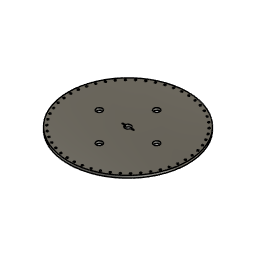
axe central v11 (Autodesk Fusion 360 design; units mm, degrees)
Autodesk Fusion 360 part; units mm, degrees
sketch "Esquisse1" plane through (0, 0, 0) normal (0, 0, 1) x (1, 0, 0)
  line L0 (-0.8543, -2.161) -> (-1.1188, -2.036)
  line L1 (1.1236, 2.043) -> (1.3703, 1.886)
  line L2 (-1.3655, -1.88) -> (-1.4051, -1.847)
  line L3 (-0.2892, -2.306) -> (-0.5764, -2.251)
  line L4 (-0.8543, 2.167) -> (-0.5764, 2.257)
  line L5 (1.4099, -1.847) -> (1.3703, -1.88)
  line L6 (-1.4051, 1.853) -> (-1.3655, 1.886)
  line L7 (1.4099, -0.321) -> (1.4099, -1.847)
  line L8 (1.3703, 1.886) -> (1.4099, 1.853)
  line L9 (-0.5764, -2.251) -> (-0.8543, -2.161)
  line L10 (-1.4051, -1.847) -> (-1.4051, -0.321)
  line L11 (0.0024, 2.331) -> (0.2941, 2.312)
  line L12 (-1.3655, 1.886) -> (-1.1188, 2.043)
  line L13 (-1.1188, 2.043) -> (-0.8543, 2.167)
  line L14 (1.4099, 1.853) -> (1.4099, 0.327)
  line L15 (4.9099, 0.327) -> (4.9099, -0.321)
  line L16 (0.0024, -2.324) -> (-0.2892, -2.306)
  line L17 (-4.9051, -0.321) -> (-4.9051, 0.327)
  line L18 (0.5813, -2.251) -> (0.2941, -2.306)
  line L19 (-0.5764, 2.257) -> (-0.2892, 2.312)
  line L20 (0.8591, 2.167) -> (1.1236, 2.043)
  line L21 (1.3703, -1.88) -> (1.1236, -2.036)
  line L22 (-1.4051, -0.321) -> (-4.9051, -0.321)
  line L23 (-1.1188, -2.036) -> (-1.3655, -1.88)
  line L24 (1.4099, 0.327) -> (4.9099, 0.327)
  line L25 (-1.4051, 0.327) -> (-1.4051, 1.853)
  line L26 (4.9099, -0.321) -> (1.4099, -0.321)
  line L27 (0.5813, 2.257) -> (0.8591, 2.167)
  line L28 (1.1236, -2.036) -> (0.8591, -2.161)
  line L29 (-0.2892, 2.312) -> (0.0024, 2.331)
  line L30 (0.2941, -2.306) -> (0.0024, -2.324)
  line L31 (-4.9051, 0.327) -> (-1.4051, 0.327)
  line L32 (0.2941, 2.312) -> (0.5813, 2.257)
  line L33 (0.8591, -2.161) -> (0.5813, -2.251)
  line L34 (-1.4051, 1.853) -> (1.4099, -1.847) construction
  line L35 (-1.4051, -1.847) -> (1.4099, 1.853) construction
  circle A0 centre (0.0024, 0.003) radius 30
  circle A1 centre (-24, 0) radius 2.5
  line L36 (0, 1.75) -> (0, 22.5)
  circle A2 centre (24, 0) radius 2.5
  circle A3 centre (-0.0006, -23.9945) radius 2.5
  circle A4 centre (-0.0006, 24.0055) radius 2.5
  circle A5 centre (0.0055, 24.0006) radius 2.5
  circle A6 centre (0.0055, -23.9994) radius 2.5
  circle A7 centre (0.0024, 0.003) radius 15
  circle A8 centre (0.0024, 0.003) radius 18
  circle A9 centre (0.0024, 0.003) radius 2.5
  circle A10 centre (0.0024, 0.003) radius 4.5
  point P0 (0.0024, 0.003)
  dimension "d1" = 60
  dimension "d3" = 5
  dimension "d6" = 180
  dimension "d7" = 30
  dimension "d9" = 3
  dimension "d32" = 5
  dimension "d33" = 2
  constraint midpoint L35 P0
  constraint coincident P0 A0.centre
  constraint symmetric A1 L36 A2
  constraint concentric A0 A7
  measures "d1" diameter of A0
  measures "d3" diameter of A1
  measures "d7" diameter of A7
  measures "d32" diameter of A9
extrude "Extrusion1" add sketch "Esquisse1" along normal blind 3 contours L0 L2 L3 L5 L7 L9 L10 L16 L18 L21 L22 L23 L26 L28 L30 L33 A9 | L22 L26 A9 A10 | L4 L6 L12 L13 L19 L25 L29 L31 L36 A9 | L31 L36 A9 A10 | L1 L8 L11 L14 L20 L24 L27 L29 L32 L36 A9 | L24 L36 A9 A10 | A0 | A7 | A8 makes body 1
extrude "Extrusion2" add sketch "Esquisse1" along normal blind 152 separate body contours A8 makes body 2
ref_plane "Plan de construction1" through (0, 0, 152) normal (0, 0, 1) x (1, 0, 0)
sketch "Esquisse4" plane through (0, 0, 152) normal (0, 0, 1) x (1, 0, 0)
  line L0 (1.3703, -1.88) -> (1.1236, -2.036)
  line L1 (1.4099, -1.847) -> (1.3703, -1.88)
  line L2 (1.4099, -0.321) -> (1.4099, -1.847)
  line L3 (4.9099, -0.321) -> (1.4099, -0.321)
  line L4 (4.9099, 0.327) -> (4.9099, -0.321)
  line L5 (1.4099, 0.327) -> (4.9099, 0.327)
  line L6 (1.4099, 1.853) -> (1.4099, 0.327)
  line L7 (1.3703, 1.886) -> (1.4099, 1.853)
  line L8 (1.1236, 2.043) -> (1.3703, 1.886)
  line L9 (0.8591, 2.167) -> (1.1236, 2.043)
  line L10 (0.5813, 2.257) -> (0.8591, 2.167)
  line L11 (0.2941, 2.312) -> (0.5813, 2.257)
  line L12 (0.0024, 2.331) -> (0.2941, 2.312)
  line L13 (-0.2892, 2.312) -> (0.0024, 2.331)
  line L14 (-0.5764, 2.257) -> (-0.2892, 2.312)
  line L15 (-0.8543, 2.167) -> (-0.5764, 2.257)
  line L16 (-1.1188, 2.043) -> (-0.8543, 2.167)
  line L17 (-1.3655, 1.886) -> (-1.1188, 2.043)
  line L18 (-1.4051, 1.853) -> (-1.3655, 1.886)
  line L19 (-1.4051, 0.327) -> (-1.4051, 1.853)
  line L20 (-4.9051, 0.327) -> (-1.4051, 0.327)
  line L21 (-4.9051, -0.321) -> (-4.9051, 0.327)
  line L22 (-1.4051, -0.321) -> (-4.9051, -0.321)
  line L23 (-1.4051, -1.847) -> (-1.4051, -0.321)
  line L24 (-1.3655, -1.88) -> (-1.4051, -1.847)
  line L25 (-1.1188, -2.036) -> (-1.3655, -1.88)
  line L26 (-0.8543, -2.161) -> (-1.1188, -2.036)
  line L27 (-0.5764, -2.251) -> (-0.8543, -2.161)
  line L28 (-0.2892, -2.306) -> (-0.5764, -2.251)
  line L29 (0.0024, -2.324) -> (-0.2892, -2.306)
  line L30 (0.2941, -2.306) -> (0.0024, -2.324)
  line L31 (0.5813, -2.251) -> (0.2941, -2.306)
  line L32 (0.8591, -2.161) -> (0.5813, -2.251)
  line L33 (1.1236, -2.036) -> (0.8591, -2.161)
  circle A0 centre (0.0024, 0.003) radius 30
  circle A1 centre (0.0024, 0.003) radius 2.5
  arc A2 (1.5758, 25.9458) -> (-1.571, 22.0602) centre (-0.0006, 24.0055) ccw
  arc A3 (-1.571, 22.0602) -> (1.5758, 25.9458) centre (0.0055, 24.0006) ccw
  arc A4 (1.5758, -22.0542) -> (-1.571, -25.9398) centre (-0.0006, -23.9945) ccw
  arc A5 (-1.571, -25.9398) -> (1.5758, -22.0542) centre (0.0055, -23.9994) ccw
  circle A6 centre (24, 0) radius 2.5
  circle A7 centre (-24, 0) radius 2.5
  dimension "d19" = 5
  constraint concentric A0 A1
  measures "d19" diameter of A1
extrude "2ieme support externe" add sketch "Esquisse1" along normal blind 5 separate body contours L0 L2 L3 L5 L7 L9 L10 L16 L18 L21 L22 L23 L26 L28 L30 L33 A9 | L0 L1 L2 L3 L4 L5 L6 L7 L8 L9 L10 L11 L12 L13 L14 L16 L18 L19 L20 L21 L22 L23 L24 L25 L26 L27 L28 L29 L30 L31 L32 L33 A9 | L22 L26 A9 A10 | L22 L31 A9 A10 | L17 L22 L31 A10 | L4 L6 L12 L13 L19 L25 L29 L31 L36 A9 | L31 L36 A9 A10 | L24 L26 A9 A10 | L15 L24 L26 A10 | L1 L8 L11 L14 L20 L24 L27 L29 L32 L36 A9 | L24 L36 A9 A10 | A0 | A7 | A8 makes body 3
extrude "Extrusion3" add sketch "Esquisse4" against normal blind 3 contours A0 | A2 A3 | A4 A5 | A6 | A7 bodies 2
extrude "Extrusion4" cut sketch "Esquisse4" against normal blind 7 contours A2 A3 | A4 A5 | A6 | A7 bodies 2
sketch "Esquisse1 (2)" plane through (0, 0, 152) normal (0, 0, 1) x (1, 0, 0) in component "disque flap"
  circle A0 centre (0, 0) radius 50
  circle A1 centre (48, 0) radius 0.75
  circle A2 centre (47.6215, 6.016) radius 0.75
  circle A3 centre (46.492, 11.9371) radius 0.75
  circle A4 centre (44.6293, 17.67) radius 0.75
  circle A5 centre (42.0627, 23.1242) radius 0.75
  circle A6 centre (38.8328, 28.2137) radius 0.75
  circle A7 centre (34.9905, 32.8583) radius 0.75
  circle A8 centre (30.5964, 36.9846) radius 0.75
  circle A9 centre (25.7197, 40.5277) radius 0.75
  circle A10 centre (20.4374, 43.4317) radius 0.75
  circle A11 centre (14.8328, 45.6507) radius 0.75
  circle A12 centre (8.9943, 47.1498) radius 0.75
  circle A13 centre (3.0139, 47.9053) radius 0.75
  circle A14 centre (-3.0139, 47.9053) radius 0.75
  circle A15 centre (-8.9943, 47.1498) radius 0.75
  circle A16 centre (-14.8328, 45.6507) radius 0.75
  circle A17 centre (-20.4374, 43.4317) radius 0.75
  circle A18 centre (-25.7197, 40.5277) radius 0.75
  circle A19 centre (-30.5964, 36.9846) radius 0.75
  circle A20 centre (-34.9905, 32.8583) radius 0.75
  circle A21 centre (-38.8328, 28.2137) radius 0.75
  circle A22 centre (-42.0627, 23.1242) radius 0.75
  circle A23 centre (-44.6293, 17.67) radius 0.75
  circle A24 centre (-46.492, 11.9371) radius 0.75
  circle A25 centre (-47.6215, 6.016) radius 0.75
  circle A26 centre (-48, 0) radius 0.75
  circle A27 centre (-47.6215, -6.016) radius 0.75
  circle A28 centre (-46.492, -11.9371) radius 0.75
  circle A29 centre (-44.6293, -17.67) radius 0.75
  circle A30 centre (-42.0627, -23.1242) radius 0.75
  circle A31 centre (-38.8328, -28.2137) radius 0.75
  circle A32 centre (-34.9905, -32.8583) radius 0.75
  circle A33 centre (-30.5964, -36.9846) radius 0.75
  circle A34 centre (-25.7197, -40.5277) radius 0.75
  circle A35 centre (-20.4374, -43.4317) radius 0.75
  circle A36 centre (-14.8328, -45.6507) radius 0.75
  circle A37 centre (-8.9943, -47.1498) radius 0.75
  circle A38 centre (-3.0139, -47.9053) radius 0.75
  circle A39 centre (3.0139, -47.9053) radius 0.75
  circle A40 centre (8.9943, -47.1498) radius 0.75
  circle A41 centre (14.8328, -45.6507) radius 0.75
  circle A42 centre (20.4374, -43.4317) radius 0.75
  circle A43 centre (25.7197, -40.5277) radius 0.75
  circle A44 centre (30.5964, -36.9846) radius 0.75
  circle A45 centre (34.9905, -32.8583) radius 0.75
  circle A46 centre (38.8328, -28.2137) radius 0.75
  circle A47 centre (42.0627, -23.1242) radius 0.75
  circle A48 centre (44.6293, -17.67) radius 0.75
  circle A49 centre (46.492, -11.9371) radius 0.75
  circle A50 centre (47.6215, -6.016) radius 0.75
  arc A51 (-1.571, 22.0602) -> (1.5758, 25.9458) centre (0.0055, 24.0006) ccw
  arc A52 (1.5758, 25.9458) -> (-1.571, 22.0602) centre (-0.0006, 24.0055) ccw
  circle A53 centre (-24, 0) radius 2.5
  circle A54 centre (24, 0) radius 2.5
  arc A55 (-1.571, -25.9398) -> (1.5758, -22.0542) centre (0.0055, -23.9994) ccw
  arc A56 (1.5758, -22.0542) -> (-1.571, -25.9398) centre (-0.0006, -23.9945) ccw
  circle A57 centre (0.0024, 0.003) radius 30
  arc A58 (-2.4765, -0.321) -> (2.4814, -0.321) centre (0.0024, 0.003) ccw
  line L0 (2.4814, -0.321) -> (4.9099, -0.321)
  line L1 (4.9099, -0.321) -> (4.9099, 0.327)
  line L2 (4.9099, 0.327) -> (2.4814, 0.327)
  arc A59 (2.4814, 0.327) -> (-2.4765, 0.327) centre (0.0024, 0.003) ccw
  line L3 (-2.4765, 0.327) -> (-4.9051, 0.327)
  line L4 (-4.9051, 0.327) -> (-4.9051, -0.321)
  line L5 (-4.9051, -0.321) -> (-2.4765, -0.321)
  dimension "d22" = 100
  dimension "d23" = 1.5
  dimension "d25" = 360
  constraint coincident A0.centre origin
  measures "d22" diameter of A0
  measures "d23" diameter of A1
extrude "Extrusion2'" add sketch "Esquisse1 (2)" along normal blind 2 separate body contours A0 | A57 makes body 4 in component "disque flap"
copy_body "Copier/Coller des corps1" bodies 4 makes body 5 in component "disque flap"
move_body "Déplacer1" bodies 5 to x (1, 0, 0) y (0, 1, 0) z (0, 0, 1) at (0, 0, -151) in component "disque flap"
extrude "Extrusion5" add sketch "Esquisse1" along normal blind 5 separate body contours L0 L2 L3 L5 L7 L9 L10 L16 L18 L21 L22 L23 L26 L28 L30 L33 A9 | L22 L26 A9 A10 | L4 L6 L12 L13 L19 L25 L29 L31 L36 A9 | L31 L36 A9 A10 | L1 L8 L11 L14 L20 L24 L27 L29 L32 L36 A9 | L24 L36 A9 A10 | A0 | A7 | A8 makes body 6
extrude "Extrusion7" add sketch "Esquisse1" along normal blind 7 separate body contours L22 L26 A9 A10 | L22 L31 A9 A10 | L31 L36 A9 A10 | L24 L26 A9 A10 | L24 L36 A9 A10 makes body 7
combine "Combiner1" operation add target body 1 tool bodies 2
move_body "Déplacer1'" bodies 3 to x (1, 0, 0) y (0, 1, 0) z (0, 0, 1) at (0, 0, -20)
move_body "Déplacer2" bodies 6 to x (1, 0, 0) y (0, 1, 0) z (0, 0, 1) at (0, 0, 165)
move_body "Déplacer3" bodies 7 to x (1, 0, 0) y (0, 1, 0) z (0, 0, 1) at (0, 0, -23)
combine "Combiner2" operation add target body 3 tool bodies 7 keep tools
hole "Perçage1" at (0, 0, -15) direction (0, 0, -1) diameter 3 depth 8 tip angle 180 counterbore diameter 6 counterbore depth 3 bodies 3 7
move_body "Déplacer2'" bodies 5 to x (1, 0, 0) y (0, 1, 0) z (0, 0, 1) at (0, 0, -10) in component "disque flap"
move_body "Déplacer3'" bodies 4 to x (1, 0, 0) y (0, 1, 0) z (0, 0, 1) at (0, 0, 5) in component "disque flap"
component "disque flap" placed x (1, 0, 0) y (0, 1, 0) z (0, 0, 1) at (0, 0, 0)
hidden bodies 1 3 6 7 4
equation "d1 = d_support"
equation "d_support = 60 mm"
equation "d3 = d_vis"
equation "d_vis = 5 mm" comment "diametre vis"
equation "d7 = d_interne_tube"
equation "d_interne_tube = 30 mm"
equation "d9 = epaisseur"
equation "epaisseur = 3 mm"
equation "d11 = epaisseur"
equation "d13 = l_axe"
equation "l_axe = 146 mm + 2 * epaisseur"
equation "d16 = l_axe"
equation "d17 = -epaisseur"
equation "d19 = d_vis"
named bodies: "shell", "externe", "top", "bottom", "support externe", "support externe 2"
